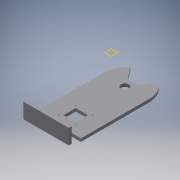
# Autodesk Inventor part: Основание
Saved by Autodesk Inventor 2018.3 (Build 223284000, 284)
## iProperties
Created: 1900-01-01
Part Number: Основание
Material: Типовые
Document SubType Name: Modeling
Designer: Leancher
Density: 1 g/cm^3
Appearance: По умолчанию
Author: Leancher
Revision Number: ANYUNSPECIFIED
Autodesk Inventor part; units mm, degrees
ref_plane "YZ Plane" through (0, 0, 0) normal (1, 0, 0) x (0, 1, 0)
ref_plane "XZ Plane" through (0, 0, 0) normal (0, 1, 0) x (-1, 0, 0)
ref_plane "XY Plane" through (0, 0, 0) normal (0, 0, 1) x (1, 0, 0)
ref_plane "РабПлоскость1" through (-120, 75, 10) normal (0, 0, 1) x (1, 0, 0)
sketch "Эскиз1" plane through (-120, 75, 10) normal (0, 0, 1) x (1, 0, 0)
  arc A0 (195, -69.7605) -> (166.6667, -11.0474) centre (120, -69.7605) ccw
  line L0 (166.6667, -11.0474) -> (141.9195, -42.1827)
  arc A1 (98.0805, -42.1827) -> (141.9195, -42.1827) centre (120, -24.7605) ccw
  line L1 (98.0805, -42.1827) -> (73.3333, -11.0474)
  arc A2 (73.3333, -11.0474) -> (45, -69.7605) centre (120, -69.7605) ccw
  line L2 (195, -69.7605) -> (195, -295.0427)
  line L3 (195, -295.0427) -> (45, -295.0427)
  line L4 (45, -295.0427) -> (45, -69.7605)
  line L5 (100, -256.9167) -> (100, -216.9167)
  line L6 (100, -256.9167) -> (140, -256.9167)
  line L7 (140, -256.9167) -> (140, -216.9167)
  line L8 (140, -216.9167) -> (100, -216.9167)
  circle A3 centre (148, -208.9167) radius 1.55
  circle A4 centre (148, -264.9167) radius 1.55
  circle A5 centre (92, -208.9167) radius 1.55
  circle A6 centre (92, -264.9167) radius 1.55
  circle A7 centre (120, -75) radius 13.15
  dimension "d21" = 26.3
  constraints: 19 end point, 8 centre point, 6 point on circle, 2 perpendicular
  measures "d21" diameter of A7
extrude "Выдавливание1" add sketch "Эскиз1" against normal blind 10
sketch "Эскиз2" plane through (-120, 75, 10) normal (0, 0, 1) x (1, 0, 0)
  line L0 (45, -324.9233) -> (44.9921, -334.9232)
  line L1 (44.9921, -334.9232) -> (194.992, -335.0427)
  line L2 (194.992, -335.0427) -> (195, -325.0427)
  line L3 (195, -325.0427) -> (45, -324.9233)
  point P0 (120, -75)
  constraints: 8 end point
extrude "Выдавливание2" add sketch "Эскиз2" along normal blind 50
